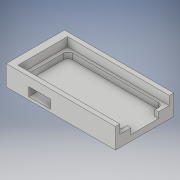
# Autodesk Inventor part: PiHolder
Saved by Autodesk Inventor 2019 (Build 230136000, 136)
## iProperties
Created: 2019-04-12
Part Number: PiHolder
Material: Generic
Document SubType Name: Modeling
Designer: Epsilon
Density: 1 g/cm^3
Appearance: Default
Author: Epsilon
Autodesk Inventor part; units mm, degrees
ref_plane "YZ Plane" through (0, 0, 0) normal (1, 0, 0) x (0, 1, 0)
ref_plane "XZ Plane" through (0, 0, 0) normal (0, 1, 0) x (-1, 0, 0)
ref_plane "XY Plane" through (0, 0, 0) normal (0, 0, 1) x (1, 0, 0)
sketch "Sketch2" plane through (0, 0, 0) normal (0, 1, 0) x (-1, 0, 0)
  line L0 (0, 0) -> (75, 0)
  line L1 (75, 0) -> (75, -40)
  line L2 (75, -40) -> (0, -40)
  line L3 (0, -40) -> (0, 0)
  dimension "d4" = 75
  dimension "d5" = 40
  constraints: 8 end point, 2 parallel, 1 horizontal, 1 perpendicular
  measures "d4" distance of L1.end L2.end
  measures "d5" distance of L0.end L1.end
extrude "Extrusion2" add sketch "Sketch2" along normal blind 14
sketch "Sketch4" plane through (0, 14, 0) normal (0, 1, 0) x (1, 0, 0)
  line L0 (0, 0) -> (0, 40) projected
  line L1 (0, 3) -> (-70, 3)
  line L2 (-70, 3) -> (-70, 37)
  line L3 (-70, 37) -> (0, 37)
  line L4 (0, 37) -> (0, 3)
  line L5 (-75, 40) -> (-75, 0) construction
  line L6 (-75, 20) -> (0, 20) construction
  dimension "d8" = 70
  dimension "d9" = 34
  constraints: 10 end point, 2 midpoint, 2 parallel, 2 perpendicular, 1 horizontal, 1 point on line, 1 other
  measures "d8" distance of L2.end L3.end
  measures "d9" distance of L1.end L2.end
extrude "Extrusion3" cut sketch "Sketch4" against normal blind 10
sketch "Sketch5" plane through (0, 4, 0) normal (0, 1, 0) x (1, 0, 0)
  line L0 (0, 3) -> (-70, 3) projected
  line L1 (-70, 37) -> (0, 37) projected
  line L2 (0, 3) -> (-70, 3)
  line L3 (-70, 3) -> (-70, 37)
  line L4 (-70, 37) -> (0, 37)
  line L5 (0, 37) -> (0, 10.475)
  line L6 (-2.5, 5) -> (-67.5, 5)
  line L7 (-67.5, 5) -> (-67.5, 35)
  line L8 (-67.5, 35) -> (-2.5, 35)
  line L9 (-2.5, 35) -> (-2.5, 29.525)
  line L10 (0, 40) -> (0, 0) construction
  line L11 (0, 20) -> (-70, 20) construction
  line L12 (-70, 3) -> (-70, 37) construction
  line L13 (-35, 3) -> (-35, 35) construction
  line L14 (0, 37) -> (0, 3) projected
  line L15 (-2.5, 10.475) -> (0, 10.475)
  line L16 (0, 29.525) -> (-2.5, 29.525)
  line L17 (-2.5, 10.475) -> (-2.5, 5)
  line L18 (0, 10.475) -> (0, 3)
  dimension "d12" = 65
  dimension "d13" = 30
  dimension "d17" = 19.05
  constraints: 28 end point, 7 parallel, 4 midpoint, 3 horizontal, 3 perpendicular, 1 point on line, 4 other
  measures "d12" distance of L7.end L8.end
  measures "d13" distance of L6.end L7.end
  measures "d17" distance of L16.start L5.end
extrude "Extrusion5" add sketch "Sketch5" along normal blind 4 contours L0 L3 L1 L5 L16 L9 L8 L7 L6 L17 L15 L14
fillet "Fillet2" radius 3 4 edges at (-2.5, 6, -5) (-67.5, 6, -5) (-67.5, 6, -35) (-2.5, 6, -35)
sketch "Sketch7" plane through (-75, 0, 0) normal (0, 0, 1) x (1, 0, 0)
  line L0 (15.4, 2) -> (30.4, 2)
  line L1 (30.4, 2) -> (30.4, 8)
  line L2 (30.4, 8) -> (15.4, 8)
  line L3 (15.4, 8) -> (15.4, 2)
  line L4 (15.4, 5) -> (30.4, 5) construction
  line L5 (22.9, 8) -> (22.9, 2) construction
  line L6 (10.5, 8) -> (10.5, 4) construction
  line L7 (10.5, 4) -> (69.5, 4) construction
  point P0 (75, 0)
  dimension "d29" = 15
  dimension "d30" = 6
  dimension "d31" = 12.4
  dimension "d32" = 2
  constraints: 12 end point, 4 midpoint, 2 parallel, 1 horizontal, 1 perpendicular
  measures "d29" distance of L2.end L1.end
  measures "d30" distance of L1.end L0.end
  measures "d31" distance between parallel lines of L5 L6
  measures "d32" distance between parallel lines of L7 L0
extrude "Extrusion7" cut sketch "Sketch7" against normal blind 6.35
body "Solid2"
